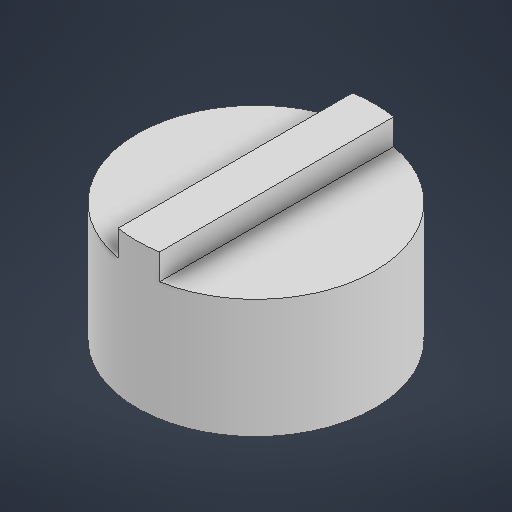
# Autodesk Inventor part: RamaKola
Saved by Autodesk Inventor 2026 (Build 300175000, 175)
## iProperties
Created: 2025-04-28
Part Number: RamaKola
Material: Generic
Document SubType Name: Modeling
Designer: isan
Density: 1 g/cm^3
Appearance: Default
Author: isan
Autodesk Inventor part; units mm, degrees
ref_plane "YZ Plane" through (0, 0, 0) normal (1, 0, 0) x (0, 1, 0)
ref_plane "XZ Plane" through (0, 0, 0) normal (0, 1, 0) x (-1, 0, 0)
ref_plane "XY Plane" through (0, 0, 0) normal (0, 0, 1) x (1, 0, 0)
sketch "Sketch1" plane through (0, 0, 0) normal (0, 0, 1) x (1, 0, 0)
  circle A0 centre (0, 0) radius 4.6
  dimension "d0" = 9.2
  constraints: 1 centre point, 1 coincident
  measures "d0" diameter of A0
extrude "Extrusion1" add sketch "Sketch1" along normal blind 4.6
sketch "Sketch2" plane through (0, 0, 0) normal (0, 0, -1) x (-1, 0, 0)
  circle A0 centre (0, 0) radius 2.6
  dimension "d3" = 5.2
  constraints: 1 centre point, 1 coincident
  measures "d3" diameter of A0
extrude "Extrusion2" cut sketch "Sketch2" against normal blind 2.6
sketch "Sketch4" plane through (0, 0, 4.6) normal (0, 0, 1) x (1, 0, 0)
  line L0 (0.8, 6.5) -> (-0.8, 6.5)
  line L1 (-0.8, 6.5) -> (-0.8, -6.5)
  line L2 (-0.8, -6.5) -> (0.8, -6.5)
  line L3 (0.8, -6.5) -> (0.8, 6.5)
  line L4 (0.8, 6.5) -> (-0.8, -6.5) construction
  line L5 (-0.8, 6.5) -> (0.8, -6.5) construction
  circle A0 centre (0, 0) radius 4.6
  circle A1 centre (0, 0) radius 4.6 projected
  point P0 (0.8, 4.5299)
  point P1 (-0.8, 4.5299)
  point P2 (-0.8, -4.5299)
  point P3 (0.8, -4.5299)
  dimension "d14" = 1.6
  dimension "d15" = 13
  constraints: 12 end point, 2 midpoint, 2 parallel, 1 centre point, 1 coincident, 1 concentric, 1 horizontal, 1 perpendicular
  measures "d14" distance of L1.end L2.end
  measures "d15" distance of L0.end L1.end
extrude "Extrusion4" add sketch "Sketch4" along normal blind 1 contours L3 A0 L1
body "Solid1"
